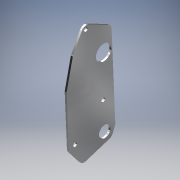
# Autodesk Inventor part: Module Plate 1
Saved by Autodesk Inventor 2019 (Build 230136000, 136)
## iProperties
Created: 2019-10-19
Part Number: Module Plate 1
Material: Aluminum 6061
Document SubType Name: Modeling
Designer: admin
Density: 2.7 g/cm^3
Appearance: Aluminum - Flat
Mass: 225.839 g
Surface Area: 449.408 cm^2
Volume: 83.6441 cm^3
Height: 70.000 mm
Author: admin
Autodesk Inventor part; units mm, degrees
ref_plane "YZ Plane" through (0, 0, 0) normal (1, 0, 0) x (0, 1, 0)
ref_plane "XZ Plane" through (0, 0, 0) normal (0, 1, 0) x (-1, 0, 0)
ref_plane "XY Plane" through (0, 0, 0) normal (0, 0, 1) x (1, 0, 0)
sketch "Sketch1" plane through (0, 0, 0) normal (1, 0, 0) x (0, 1, 0)
  circle A0 centre (0, 0) radius 62.5 construction
  circle A1 centre (-146.0656, -2.5) radius 50 construction
  line L0 (-146.0656, -2.5) -> (0, 0) construction
  line L1 (-172.7208, -52.5) -> (-113.4241, -52.5) construction
  line L2 (-16.0459, -62.5) -> (40.9165, -62.5) construction
  line L3 (-162.86, -17.263) -> (-144.3319, -24.7934)
  line L4 (-144.3319, -24.7934) -> (-74.6779, -21.7515)
  line L5 (42.063, -16.6532) -> (72.2375, 41.3128)
  line L6 (72.2375, 41.3128) -> (-2.0558, 79.9865)
  line L7 (-2.0558, 79.9865) -> (-145.8225, 73.708)
  line L8 (-145.8225, 73.708) -> (-182.9035, 44.86)
  line L9 (-182.9035, 44.86) -> (-162.86, -17.263)
  circle A2 centre (0, 0) radius 16.3
  circle A3 centre (-146.0656, -2.5) radius 12.2
  line L10 (-153.5959, -21.0282) -> (-146.0656, -2.5) construction
  arc A4 (-63.375, -21.2579) -> (-74.6779, -21.7515) centre (-69.3319, -14.5113) ccw construction
  line L11 (-99.9551, -22.8554) -> (-99.3168, -22.8275) construction
  line L12 (-99.3168, -22.8275) -> (-63.375, -21.2579) construction
  line L13 (-63.375, -21.2579) -> (-99.9551, -22.8554) construction
  line L14 (-74.6779, -21.7515) -> (42.063, -16.6532)
  line L15 (0, 0) -> (-212.6616, 0) construction
  circle A5 centre (-86.0656, 0.7731) radius 4.25
  dimension "d0" = 125
  dimension "d1" = 100
  dimension "d2" = 146.087
  dimension "d3" = 10
  dimension "d4" = 20
  dimension "d5" = 32.6
  dimension "d6" = 24.4
  dimension "d7" = 23.099
  dimension "d8" = 20
  dimension "d9" = 130
  dimension "d10" = 110
  dimension "d12" = 155.381
  dimension "d13" = 80
  dimension "d14" = 90
  dimension "d15" = 150
  dimension "Height" = 70
  dimension "d17" = 45
  dimension "d18" = 60
  dimension "d30" = 8.5
  dimension "d31" = 23
  dimension "d32" = 60
  constraints: 32 end point, 6 centre point, 5 parallel, 4 point on line, 3 coincident, 3 horizontal, 2 point on circle, 2 tangent, 1 midpoint, 1 perpendicular
  measures "d0" diameter of A0
  measures "d1" diameter of A1
  measures "d2" distance of L0.start L0.end
  measures "d3" distance between parallel lines of L2 L1
  measures "d4" distance from line of L0.start L3
  measures "d5" diameter of A2
  measures "d6" diameter of A3
  measures "d7" angle of L0 L3
  measures "d8" distance of L3.start L3.end
  measures "d9" angle of L3 L9
  measures "d10" angle of L9 L8
  measures "d12" angle of L4 L3
  measures "d13" distance from line of L15.start L7
  measures "d14" angle of L5 L6
  measures "d15" angle of L7 L6
  measures "Height" distance from line of point (0, 0) L6
  measures "d17" distance from line of L15.start L5
  measures "d18" distance from line of L10.end L8
  measures "d30" diameter of A5
  measures "d31" distance from line of L4 A5.centre
  measures "d32" horizontal distance of L0.start A5.centre
extrude "Extrusion1" add sketch "Sketch1" along normal blind 4
fillet "Fillet3" radius 10 6 edges at (2, 72.2375, 41.3128) (2, 42.063, -16.6532) (2, -144.3319, -24.7934) (2, -162.86, -17.263) (2, -182.9035, 44.86) (2, -145.8225, 73.708)
chamfer "Chamfer1" distance 32 angle 45 1 edges at (2, -2.0558, 79.9865)
fillet "Fillet4" radius 10 2 edges at (2, 26.3287, 65.2108) (2, -34.0253, 78.5903)
sketch "Sketch2" plane through (4, 0, 0) normal (1, 0, 0) x (0, 0, -1)
  circle A0 centre (0, 0) radius 16.3
  circle A1 centre (0, 0) radius 16.3 projected
  circle A2 centre (-60.3803, -138.5253) radius 4.25
  line L0 (-71.7494, -148.34) -> (-49.1595, -177.377) projected
  line L1 (-38.1961, -180.7535) -> (12.8252, -164.2919) projected
  circle A3 centre (-37.9106, 61.4474) radius 4.25
  arc A4 (-32.4427, 67.6201) -> (-45.9302, 63.3673) centre (-37.0601, 58.7499) ccw projected
  line L2 (11.532, 44.7289) -> (-32.4427, 67.6201) projected
  line L3 (-45.9302, 63.3673) -> (-64.6029, 27.4965) projected
  point P0 (18.0192, 10.7846)
  point P1 (18.8908, -9.1727)
  dimension "d39" = 32.6
  dimension "d42" = 8.5
  dimension "d43" = 15
  dimension "d44" = 47
  dimension "d45" = 8.5
  dimension "d47" = 8
  dimension "d48" = 8
  constraints: 3 centre point, 2 other
  measures "d39" diameter of A0
  measures "d42" diameter of A2
  measures "d43" distance from line of L0 A2.centre
  measures "d44" distance from line of L1 A2.centre
  measures "d45" diameter of A3
  measures "d47" distance from line of L2 A3.centre
  measures "d48" distance from line of L3 A3.centre
extrude "Extrusion2" cut sketch "Sketch2" against normal blind 9.5
body "Solid1"
